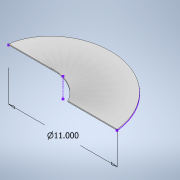
# Autodesk Inventor part: rampLowerHalf
Saved by Autodesk Inventor 2020 (Build 240168000, 168)
## iProperties
Created: 2021-03-23
Part Number: rampLowerHalf
Material: Generic
Document SubType Name: Modeling
Designer: tdmp4
Density: 1 g/cm^3
Appearance: Default
Author: tdmp4
Autodesk Inventor part; units mm, degrees
ref_plane "YZ Plane" through (0, 0, 0) normal (1, 0, 0) x (0, 1, 0)
ref_plane "XZ Plane" through (0, 0, 0) normal (0, 1, 0) x (-1, 0, 0)
ref_plane "XY Plane" through (0, 0, 0) normal (0, 0, 1) x (1, 0, 0)
sketch "Sketch6" plane through (0, 0, 0) normal (0, 0, 1) x (1, 0, 0)
  line L0 (139.7, -0.0309) -> (12.7, -0.0309)
  line L1 (12.7, -0.0309) -> (12.7, 2.5091)
  line L2 (12.7, 2.5091) -> (139.7, 2.5091)
  line L3 (139.7, 2.5091) -> (139.7, -0.0309)
  point P0 (0, 0)
  dimension "d11" = 127
  dimension "d12" = 2.54
  constraints: 8 end point, 2 parallel, 1 horizontal, 1 perpendicular
  measures "d11" distance of L1.end L2.end
  measures "d12" distance of L0.end L1.end
sketch3d "3D Sketch2"
  helix H0 starts at (139.7, 0, 0) axis through (0, 0, 0) along (0, 1, 0) pitch 101.6 turns 0.5 hand right
sweep "Sweep1" add profiles "Sketch6" path "3D Sketch2"
body "Solid1"
